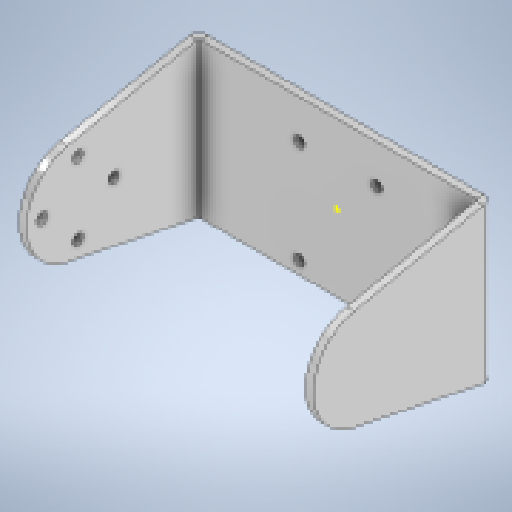
# Autodesk Inventor part: axis_14_bottom_frame
Saved by Autodesk Inventor 2026.1 (Build 301233020, 233B)
## iProperties
Created: 2023-10-27
Part Number: axis_14_bottom_frame
Material: Aluminum 6061-AHC
Document SubType Name: Sheet Metal
Designer: chanh
Density: 2.7 g/cm^3
Sheet Metal Rule: Default_mm
Appearance: Aluminum - Dark
Flat Pattern Width: 3 cm
Flat Pattern Length: 12.1659 cm
Flat Pattern Area: 36.4976 cm^2
Sheet Metal Width: 30.000 mm
Sheet Metal Length: 121.659 mm
Sheet Metal Area: 3649.757 mm^2
Author: chanh
Autodesk Inventor part; units mm, degrees
ref_plane "YZ Plane" through (0, 0, 0) normal (1, 0, 0) x (0, 1, 0)
ref_plane "XZ Plane" through (0, 0, 0) normal (0, 1, 0) x (-1, 0, 0)
ref_plane "XY Plane" through (0, 0, 0) normal (0, 0, 1) x (1, 0, 0)
sketch "Sketch1" plane through (0, 0, 0) normal (0, 0, 1) x (1, 0, 0)
  line L0 (-28.59, -15) -> (28.59, -15)
  line L1 (28.59, -15) -> (28.59, 15)
  line L2 (28.59, 15) -> (-28.59, 15)
  line L3 (-28.59, 15) -> (-28.59, -15)
  line L4 (-28.59, -15) -> (28.59, 15) construction
  line L5 (28.59, -15) -> (-28.59, 15) construction
  point P0 (0, 0)
  dimension "d0" = 57.18
  dimension "d1" = 30
  measures "d0" distance of L2.end L1.end
  measures "d1" distance of L1.end L0.end
extrude "Plate1" add sketch "Sketch1" along normal blind 1.5
sketch "Sketch2" plane through (-27.09, -15, 0) normal (-1, 0, 0) x (0, -1, 0)
  line L0 (-30, 0) -> (0, 0)
  line L1 (0, 0) -> (0, 40)
  line L2 (0, 40) -> (-30, 40)
  line L3 (-30, 40) -> (-30, 0)
  constraints: 6 end point, 1 horizontal, 1 perpendicular, 1 vertical
edge flange "Flange1" height 40 angle 90 thickness 1.5 bend radius 0.31 thickness toward (-1, 0, 0) relief tear relief width 1.5 relief depth 0.75 corner gap 0.31 corner form 0 edges at (-28.59, 0, 1.5) (28.59, 0, 1.5) wall of the first edge with corners at (-27.09, 15, 0) (-27.09, -15, 0) (-27.09, -15, 40) (-27.09, 15, 40)
bend "Bend1"
corner "Corner1"
sketch "Sketch3" plane through (28.59, -15, 40) normal (1, 0, 0) x (0, 0, -1)
  circle A0 centre (15, 15) radius 9.96
  line L0 (0, 30) -> (38.19, 30) projected
  line L1 (38.19, 0) -> (0, 0) projected
  line L2 (38.19, 30) -> (12.9705, 24.751)
  line L3 (38.19, 0) -> (12.9705, 5.249)
  line L4 (0, 30) -> (0, 0)
  point P0 (40, 15)
  dimension "d13" = 19.92
  dimension "d14" = 0
  dimension "d15" = 25
  constraints: 6 end point, 2 point on circle, 2 point on line, 2 tangent, 1 centre point, 1 horizontal alignment, 1 vertical, 1 vertical alignment
  measures "d13" diameter of A0
  measures "d14" distance of L0.end L2.start
  measures "d15" distance of point (40, 15) A0.centre
sketch "Sketch19" plane through (0, 0, 1.5) normal (0, 0, 1) x (1, 0, 0)
  point P0 (0, 0)
sketch "Sketch21" plane through (-28.59, -15, 1.81) normal (-1, 0, 0) x (0, 0, 1)
  point P0 (-1.81, 15)
sketch "Sketch23" plane through (-28.59, -15, 1.81) normal (-1, 0, 0) x (0, 0, 1)
  point P0 (-1.81, 15)
sketch "Sketch25" plane through (0, 0, 1.5) normal (0, 0, 1) x (1, 0, 0)
  circle A0 centre (7.525, 7.5) radius 0.7835
  circle A1 centre (7.525, -12.5) radius 0.7835
  circle A2 centre (-7.525, -12.5) radius 0.7835
  circle A3 centre (-7.525, 7.5) radius 0.7835
  point P0 (0, 0)
  constraints: 4 centre point, 8 other
hole "Hole12" at (7.525, 7.5, 1.5) at (7.525, -12.5, 1.5) at (-7.525, 7.5, 1.5) at (-7.525, -12.5, 1.5) direction (0, 0, -1) diameter 2.1 depth 1.5
extrude "Cut7" cut sketch "Sketch3" against normal blind 1.5 contours A0 L3 L1 L4 L0 L2
mirror "Mirror1" about plane through (0, 0, 0) normal (1, 0, 0) of "Cut7"
sketch "Sketch26" plane through (-28.59, -15, 1.81) normal (-1, 0, 0) x (0, 0, 1)
  circle A0 centre (30.19, 15) radius 0.7835 projected
  circle A1 centre (23.19, 22) radius 0.7835 projected
  circle A2 centre (23.19, 8) radius 0.7835 projected
  circle A3 centre (16.19, 15) radius 0.7835 projected
  point P0 (-1.81, 15)
hole "Hole13" at (-28.59, 0, 32) at (-28.59, 7, 25) at (-28.59, -7, 25) at (-28.59, 0, 18) direction (1, 0, 0) diameter 2.1 depth 1.5
sketch "Sketch27" plane through (-28.59, -15, 1.81) normal (-1, 0, 0) x (0, 0, 1)
  circle A0 centre (23.19, 15) radius 3 projected
  point P0 (-1.81, 15)
hole "Hole14" at (-28.59, 0, 25) direction (1, 0, 0) diameter 7.2 depth 1.5
sketch "Sketch28" plane through (28.59, -15, 1.81) normal (1, 0, 0) x (0, 0, -1)
  circle A0 centre (-30.19, 15) radius 0.7835 projected
  circle A1 centre (-23.19, 8) radius 0.7835 projected
  circle A2 centre (-23.19, 22) radius 0.7835 projected
  circle A3 centre (-16.19, 15) radius 0.7835 projected
  point P0 (1.81, 15)
hole "Hole15" at (28.59, 0, 32) at (28.59, -7, 25) at (28.59, 0, 18) at (28.59, 7, 25) direction (-1, 0, 0) diameter 2.1 depth 1.5
sketch "Sketch29" plane through (28.59, -15, 1.81) normal (1, 0, 0) x (0, 0, -1)
  circle A0 centre (-23.19, 15) radius 1.75 projected
  point P0 (1.81, 15)
hole "Hole16" at (28.59, 0, 25) direction (-1, 0, 0) diameter 5.2 depth 1.5
equation "\"d125\" = Thickness"
equation "\"d127\" = Thickness"
equation "\"d134\" = Thickness"
equation "\"d141\" = Thickness"
equation "\"d148\" = Thickness"
equation "\"d155\" = Thickness"
equation "\"d2\" = Thickness"
equation "\"d3\" = BendReliefWidth"
equation "\"d4\" = BendReliefDepth"
equation "\"d5\" = MinimumRemnant"
equation "\"d6\" = TransitionRadius"
equation "\"d9\" = BendRadius"
equation "\"d10\" = CornerReliefSize"
equation "\"d11\" = GapSize"
equation "\"d12\" = JacobiRadiusSize"
equation "\"BendReliefWidth\" = Thickness"
equation "\"BendReliefDepth\" = 0.5 * Thickness"
equation "\"CornerReliefSize\" = 4 * Thickness"
equation "\"MinimumRemnant\" = 2 * Thickness"
equation "\"TransitionRadius\" = BendRadius"
equation "\"JacobiRadiusSize\" = BendRadius"
equation "\"GapSize\" = Thickness"
equation "\"Thickness\" = 1.5"
equation "\"BendRadius\" = 0.31"
body "Solid1"
